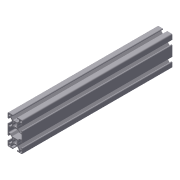
# Autodesk Inventor part: 30x60x2 in
Saved by Autodesk Inventor 2013 (Build 170138000, 138)
## iProperties
Created: 2011-07-21
Part Number: 30x60x2 in
Document SubType Name: Modeling
Designer: Dan Niemitalo
Density: 2.71 g/cm^3
Material: Aluminum-6061
Mass: 75.8168 g
Surface Area: 296.17 cm^2
Volume: 27.9767 cm^3
Author: Dan Niemitalo
Autodesk Inventor part; units mm, degrees
ref_plane "YZ Plane" through (0, 0, 0) normal (1, 0, 0) x (0, 1, 0)
ref_plane "XZ Plane" through (0, 0, 0) normal (0, 1, 0) x (-1, 0, 0)
ref_plane "XY Plane" through (0, 0, 0) normal (0, 0, 1) x (1, 0, 0)
sketch "3060" plane through (0, 0, 0) normal (0, 0, 1) x (1, 0, 0)
  line L0 (-0.1, 57.8) -> (3.3, 57.8)
  line L1 (-0.2, 59.8) -> (-0.2, 59.7)
  line L2 (-0.4, 59.5) -> (-0.5, 59.5)
  arc A0 (0, 60) -> (-0.2, 59.8) centre (0, 59.8) ccw
  arc A1 (-0.4, 59.5) -> (-0.2, 59.7) centre (-0.4, 59.7) ccw
  arc A2 (-0.5, 59.5) -> (-0.7, 59.3) centre (-0.5, 59.3) ccw
  line L3 (-0.7, 59.3) -> (-0.7, 58.4)
  arc A3 (-0.7, 58.4) -> (-0.1, 57.8) centre (-0.1, 58.4) ccw
  line L4 (-19.05, 49.05) -> (-18.15, 49.05)
  arc A4 (-19.25, 49.25) -> (-19.05, 49.05) centre (-19.05, 49.25) ccw
  line L5 (-19.25, 49.35) -> (-19.25, 49.25)
  arc A5 (-18.15, 49.05) -> (-17.55, 49.65) centre (-18.15, 49.65) ccw
  arc A6 (-19.25, 49.35) -> (-19.45, 49.55) centre (-19.45, 49.35) ccw
  line L6 (-19.55, 49.55) -> (-19.45, 49.55)
  arc A7 (-19.75, 49.75) -> (-19.55, 49.55) centre (-19.55, 49.75) ccw
  arc A8 (-17.35, 53.25) -> (-17.55, 53.05) centre (-17.35, 53.05) ccw
  line L7 (-17.35, 53.25) -> (-14.8828, 53.25)
  arc A9 (-18.45, 55.5) -> (-17.45, 54.5) centre (-17.45, 55.5) ccw
  line L8 (-19.75, 58) -> (-19.75, 49.75)
  line L9 (-17.55, 49.65) -> (-17.55, 53.05)
  arc A10 (-6.3501, 41.7194) -> (-3.1499, 41.7194) centre (-4.75, 45) ccw
  line L10 (0.5997, 38.4955) -> (-10.0997, 38.4955)
  arc A11 (-1.4694, 43.3999) -> (-1.4694, 46.6001) centre (-4.75, 45) ccw
  line L11 (-3.1499, 41.7194) -> (-1.5953, 40.4947)
  arc A12 (-1.5953, 40.4947) -> (-0.2316, 41.8641) centre (-4.75, 45) ccw
  line L12 (-0.2316, 41.8641) -> (-1.4694, 43.3999)
  line L13 (1.2545, 40.8784) -> (1.2545, 44.1)
  arc A13 (1.2545, 40.8784) -> (1.313, 40.737) centre (1.4545, 40.8784) ccw
  line L14 (-7.9047, 40.4947) -> (-6.3501, 41.7194)
  arc A14 (-9.2684, 41.8641) -> (-7.9047, 40.4947) centre (-4.75, 45) ccw
  line L15 (-8.0306, 43.3999) -> (-9.2684, 41.8641)
  arc A15 (-8.0306, 46.6001) -> (-8.0306, 43.3999) centre (-4.75, 45) ccw
  line L16 (-10.7545, 44.1) -> (-10.7545, 40.8784)
  arc A16 (-10.2926, 44.9) -> (-10.2926, 45.1) centre (-10.4658, 45) ccw
  line L17 (-10.2926, 44.9) -> (-10.7545, 44.1)
  arc A17 (-3.1499, 48.2806) -> (-6.3501, 48.2806) centre (-4.75, 45) ccw
  line L18 (-6.3501, 48.2806) -> (-7.9047, 49.5053)
  line L19 (-9.2684, 48.1359) -> (-8.0306, 46.6001)
  line L20 (-5.65, 51) -> (-8.8672, 51)
  arc A18 (-7.9047, 49.5053) -> (-9.2684, 48.1359) centre (-4.75, 45) ccw
  line L21 (-10.7545, 49.1216) -> (-10.7545, 45.9)
  arc A19 (-10.7545, 49.1216) -> (-10.813, 49.263) centre (-10.9545, 49.1216) ccw
  line L22 (-10.7545, 45.9) -> (-10.2926, 45.1)
  arc A20 (-0.2316, 48.1359) -> (-1.5953, 49.5053) centre (-4.75, 45) ccw
  line L23 (-1.4694, 46.6001) -> (-0.2316, 48.1359)
  arc A21 (-0.6328, 51) -> (-0.4914, 51.0586) centre (-0.6328, 51.2) ccw
  arc A22 (1.313, 49.263) -> (1.2545, 49.1216) centre (1.4545, 49.1216) ccw
  line L24 (1.313, 49.263) -> (5.2414, 53.1914)
  line L25 (3.4414, 54.9914) -> (-0.4914, 51.0586)
  arc A23 (-14.7414, 53.1914) -> (-14.8828, 53.25) centre (-14.8828, 53.05) ccw
  line L26 (-14.7414, 53.1914) -> (-10.813, 49.263)
  arc A24 (-13, 55.1328) -> (-12.9414, 54.9914) centre (-12.8, 55.1328) ccw
  arc A25 (-9.0086, 51.0586) -> (-8.8672, 51) centre (-8.8672, 51.2) ccw
  line L27 (-9.0086, 51.0586) -> (-12.9414, 54.9914)
  line L28 (-13, 55.1328) -> (-13, 57.6)
  arc A26 (-12.8, 57.8) -> (-13, 57.6) centre (-12.8, 57.6) ccw
  line L29 (-14.25, 55.5) -> (-14.25, 57.7)
  line L30 (-18.45, 57.7) -> (-18.45, 55.5)
  arc A27 (-17.45, 58.7) -> (-18.45, 57.7) centre (-17.45, 57.7) ccw
  arc A28 (-17.75, 60) -> (-19.75, 58) centre (-17.75, 58) ccw
  line L31 (-15.25, 58.7) -> (-17.45, 58.7)
  arc A29 (-14.25, 57.7) -> (-15.25, 58.7) centre (-15.25, 57.7) ccw
  line L32 (-12.8, 57.8) -> (-9.4, 57.8)
  arc A30 (-15.25, 54.5) -> (-14.25, 55.5) centre (-15.25, 55.5) ccw
  arc A31 (-9.4, 57.8) -> (-8.8, 58.4) centre (-9.4, 58.4) ccw
  line L33 (-9.5, 60) -> (-17.75, 60)
  line L34 (-9, 59.5) -> (-9.1, 59.5)
  line L35 (-8.8, 58.4) -> (-8.8, 59.3)
  arc A32 (-8.8, 59.3) -> (-9, 59.5) centre (-9, 59.3) ccw
  arc A33 (-9.3, 59.7) -> (-9.1, 59.5) centre (-9.1, 59.7) ccw
  line L36 (-9.3, 59.7) -> (-9.3, 59.8)
  arc A34 (-9.3, 59.8) -> (-9.5, 60) centre (-9.5, 59.8) ccw
  line L37 (-17.45, 54.5) -> (-15.25, 54.5)
  arc A35 (8.05, 53.05) -> (7.85, 53.25) centre (7.85, 53.05) ccw
  line L38 (8.05, 53.05) -> (8.05, 49.65)
  line L39 (10.25, 49.75) -> (10.25, 58)
  arc A36 (8.05, 49.65) -> (8.65, 49.05) centre (8.65, 49.65) ccw
  line L40 (8.65, 49.05) -> (9.55, 49.05)
  line L41 (9.75, 49.25) -> (9.75, 49.35)
  arc A37 (9.95, 49.55) -> (9.75, 49.35) centre (9.95, 49.35) ccw
  arc A38 (9.55, 49.05) -> (9.75, 49.25) centre (9.55, 49.25) ccw
  arc A39 (10.05, 49.55) -> (10.25, 49.75) centre (10.05, 49.75) ccw
  line L42 (9.95, 49.55) -> (10.05, 49.55)
  line L43 (5.75, 54.5) -> (7.95, 54.5)
  line L44 (7.95, 58.7) -> (5.75, 58.7)
  arc A40 (7.95, 54.5) -> (8.95, 55.5) centre (7.95, 55.5) ccw
  line L45 (8.95, 55.5) -> (8.95, 57.7)
  arc A41 (8.95, 57.7) -> (7.95, 58.7) centre (7.95, 57.7) ccw
  arc A42 (10.25, 58) -> (8.25, 60) centre (8.25, 58) ccw
  line L46 (8.25, 60) -> (0, 60)
  arc A43 (3.5, 57.6) -> (3.3, 57.8) centre (3.3, 57.6) ccw
  line L47 (3.5, 57.6) -> (3.5, 55.1328)
  arc A44 (3.4414, 54.9914) -> (3.5, 55.1328) centre (3.3, 55.1328) ccw
  arc A45 (5.75, 58.7) -> (4.75, 57.7) centre (5.75, 57.7) ccw
  line L48 (4.75, 57.7) -> (4.75, 55.5)
  arc A46 (4.75, 55.5) -> (5.75, 54.5) centre (5.75, 55.5) ccw
  arc A47 (5.3828, 53.25) -> (5.2414, 53.1914) centre (5.3828, 53.05) ccw
  line L49 (5.3828, 53.25) -> (7.85, 53.25)
  line L50 (1.2545, 44.1) -> (0.7926, 44.9)
  arc A48 (0.7926, 45.1) -> (0.7926, 44.9) centre (0.9658, 45) ccw
  line L51 (-4.8519, 50.5392) -> (-5.65, 51)
  arc A49 (-4.8519, 50.5392) -> (-4.6481, 50.5392) centre (-4.75, 50.7158) ccw
  line L52 (-3.85, 51) -> (-4.6481, 50.5392)
  line L53 (-1.5953, 49.5053) -> (-3.1499, 48.2806)
  line L54 (-0.6328, 51) -> (-3.85, 51)
  line L55 (1.2545, 45.9) -> (1.2545, 49.1216)
  line L56 (0.7926, 45.1) -> (1.2545, 45.9)
  arc A50 (-14.25, 4.5) -> (-15.25, 5.5) centre (-15.25, 4.5) ccw
  arc A51 (-14.8828, 6.75) -> (-14.7414, 6.8086) centre (-14.8828, 6.95) ccw
  line L57 (-15.25, 5.5) -> (-17.45, 5.5)
  line L58 (-14.8828, 6.75) -> (-17.35, 6.75)
  arc A52 (-19.75, 2) -> (-17.75, 0) centre (-17.75, 2) ccw
  arc A53 (-18.45, 2.3) -> (-17.45, 1.3) centre (-17.45, 2.3) ccw
  line L59 (-18.45, 4.5) -> (-18.45, 2.3)
  arc A54 (-17.45, 5.5) -> (-18.45, 4.5) centre (-17.45, 4.5) ccw
  arc A55 (-17.55, 6.95) -> (-17.35, 6.75) centre (-17.35, 6.95) ccw
  line L60 (-17.55, 6.95) -> (-17.55, 10.35)
  line L61 (-19.75, 10.25) -> (-19.75, 2)
  line L62 (0.7926, 15.1) -> (1.2545, 15.9)
  arc A56 (0.7926, 15.1) -> (0.7926, 14.9) centre (0.9658, 15) ccw
  line L63 (1.2545, 14.1) -> (0.7926, 14.9)
  line L64 (1.2545, 10.8784) -> (1.2545, 14.1)
  arc A57 (1.2545, 10.8784) -> (1.313, 10.737) centre (1.4545, 10.8784) ccw
  arc A58 (5.75, 5.5) -> (4.75, 4.5) centre (5.75, 4.5) ccw
  arc A59 (-0.4914, 8.9414) -> (-0.6328, 9) centre (-0.6328, 8.8) ccw
  line L65 (-0.4914, 8.9414) -> (3.4414, 5.0086)
  arc A60 (5.2414, 6.8086) -> (5.3828, 6.75) centre (5.3828, 6.95) ccw
  line L66 (7.95, 5.5) -> (5.75, 5.5)
  line L67 (7.85, 6.75) -> (5.3828, 6.75)
  line L68 (5.2414, 6.8086) -> (1.313, 10.737)
  arc A61 (3.5, 4.8672) -> (3.4414, 5.0086) centre (3.3, 4.8672) ccw
  line L69 (3.5, 4.8672) -> (3.5, 2.4)
  line L70 (0, 0) -> (8.25, 0)
  arc A62 (3.3, 2.2) -> (3.5, 2.4) centre (3.3, 2.4) ccw
  line L71 (3.3, 2.2) -> (-0.1, 2.2)
  arc A63 (-18.15, 19.05) -> (-17.55, 19.65) centre (-18.15, 19.65) ccw
  line L72 (-17.55, 19.65) -> (-17.55, 23.05)
  line L73 (-17.35, 23.25) -> (-14.8828, 23.25)
  arc A64 (-14.7414, 23.1914) -> (-14.8828, 23.25) centre (-14.8828, 23.05) ccw
  line L74 (-16.6, 24.9) -> (-14.7379, 24.9)
  line L75 (-14.7414, 23.1914) -> (-10.813, 19.263)
  arc A65 (-11.1604, 21.9438) -> (-10.0997, 21.5045) centre (-10.0997, 23.0045) ccw
  line L76 (-13.6772, 24.4607) -> (-11.1604, 21.9438)
  arc A66 (-13.6772, 24.4607) -> (-14.7379, 24.9) centre (-14.7379, 23.4) ccw
  arc A67 (-18.1, 26.4) -> (-16.6, 24.9) centre (-16.6, 26.4) ccw
  arc A68 (-17.35, 23.25) -> (-17.55, 23.05) centre (-17.35, 23.05) ccw
  arc A69 (-16.6, 35.1) -> (-18.1, 33.6) centre (-16.6, 33.6) ccw
  line L77 (-14.7379, 35.1) -> (-16.6, 35.1)
  arc A70 (-14.7379, 35.1) -> (-13.6772, 35.5393) centre (-14.7379, 36.6) ccw
  line L78 (-14.8828, 36.75) -> (-17.35, 36.75)
  arc A71 (-17.55, 36.95) -> (-17.35, 36.75) centre (-17.35, 36.95) ccw
  arc A72 (-14.8828, 36.75) -> (-14.7414, 36.8086) centre (-14.8828, 36.95) ccw
  line L79 (-11.1604, 38.0562) -> (-13.6772, 35.5393)
  arc A73 (-10.0997, 38.4955) -> (-11.1604, 38.0562) centre (-10.0997, 36.9955) ccw
  line L80 (-10.813, 40.737) -> (-14.7414, 36.8086)
  arc A74 (-10.813, 40.737) -> (-10.7545, 40.8784) centre (-10.9545, 40.8784) ccw
  arc A75 (-12.9414, 5.0086) -> (-13, 4.8672) centre (-12.8, 4.8672) ccw
  line L81 (-12.9414, 5.0086) -> (-9.0086, 8.9414)
  line L82 (-10.813, 10.737) -> (-14.7414, 6.8086)
  arc A76 (-10.813, 10.737) -> (-10.7545, 10.8784) centre (-10.9545, 10.8784) ccw
  line L83 (-14.25, 2.3) -> (-14.25, 4.5)
  line L84 (-13, 2.4) -> (-13, 4.8672)
  arc A77 (-13, 2.4) -> (-12.8, 2.2) centre (-12.8, 2.4) ccw
  line L85 (-19.45, 40.45) -> (-19.55, 40.45)
  arc A78 (-19.55, 40.45) -> (-19.75, 40.25) centre (-19.55, 40.25) ccw
  arc A79 (-17.55, 40.35) -> (-18.15, 40.95) centre (-18.15, 40.35) ccw
  arc A80 (-19.45, 40.45) -> (-19.25, 40.65) centre (-19.45, 40.65) ccw
  line L86 (-19.25, 40.75) -> (-19.25, 40.65)
  line L87 (-18.15, 40.95) -> (-19.05, 40.95)
  arc A81 (-19.05, 40.95) -> (-19.25, 40.75) centre (-19.05, 40.75) ccw
  line L88 (-17.55, 36.95) -> (-17.55, 40.35)
  arc A82 (10.25, 40.25) -> (10.05, 40.45) centre (10.05, 40.25) ccw
  line L89 (10.05, 40.45) -> (9.95, 40.45)
  line L90 (5.2414, 36.8086) -> (1.313, 40.737)
  line L91 (8.05, 40.35) -> (8.05, 36.95)
  arc A83 (8.65, 40.95) -> (8.05, 40.35) centre (8.65, 40.35) ccw
  line L92 (9.75, 40.65) -> (9.75, 40.75)
  line L93 (9.55, 40.95) -> (8.65, 40.95)
  arc A84 (9.75, 40.65) -> (9.95, 40.45) centre (9.95, 40.65) ccw
  arc A85 (9.75, 40.75) -> (9.55, 40.95) centre (9.55, 40.75) ccw
  arc A86 (7.1, 24.9) -> (8.6, 26.4) centre (7.1, 26.4) ccw
  line L94 (5.2379, 24.9) -> (7.1, 24.9)
  arc A87 (5.2379, 24.9) -> (4.1772, 24.4607) centre (5.2379, 23.4) ccw
  line L95 (5.3828, 23.25) -> (7.85, 23.25)
  arc A88 (5.3828, 23.25) -> (5.2414, 23.1914) centre (5.3828, 23.05) ccw
  arc A89 (8.05, 23.05) -> (7.85, 23.25) centre (7.85, 23.05) ccw
  line L96 (1.6604, 21.9438) -> (4.1772, 24.4607)
  arc A90 (0.5997, 21.5045) -> (1.6604, 21.9438) centre (0.5997, 23.0045) ccw
  line L97 (8.05, 23.05) -> (8.05, 19.65)
  line L98 (1.313, 19.263) -> (5.2414, 23.1914)
  arc A91 (1.313, 19.263) -> (1.2545, 19.1216) centre (1.4545, 19.1216) ccw
  arc A92 (8.05, 19.65) -> (8.65, 19.05) centre (8.65, 19.65) ccw
  line L99 (9.95, 19.55) -> (10.05, 19.55)
  arc A93 (10.05, 19.55) -> (10.25, 19.75) centre (10.05, 19.75) ccw
  arc A94 (9.95, 19.55) -> (9.75, 19.35) centre (9.95, 19.35) ccw
  line L100 (9.75, 19.25) -> (9.75, 19.35)
  arc A95 (9.55, 19.05) -> (9.75, 19.25) centre (9.55, 19.25) ccw
  line L101 (8.65, 19.05) -> (9.55, 19.05)
  line L102 (1.2545, 15.9) -> (1.2545, 19.1216)
  line L103 (-1.5953, 19.5053) -> (-3.1499, 18.2806)
  arc A96 (-0.2316, 18.1359) -> (-1.5953, 19.5053) centre (-4.75, 15) ccw
  arc A97 (-3.1499, 18.2806) -> (-6.3501, 18.2806) centre (-4.75, 15) ccw
  line L104 (-10.0997, 21.5045) -> (0.5997, 21.5045)
  line L105 (-1.4694, 16.6001) -> (-0.2316, 18.1359)
  line L106 (-19.75, 40.25) -> (-19.75, 19.75)
  line L107 (-18.1, 33.6) -> (-18.1, 26.4)
  arc A98 (-10.2926, 14.9) -> (-10.2926, 15.1) centre (-10.4658, 15) ccw
  line L108 (-19.05, 19.05) -> (-18.15, 19.05)
  line L109 (-19.25, 19.35) -> (-19.25, 19.25)
  arc A99 (-19.25, 19.35) -> (-19.45, 19.55) centre (-19.45, 19.35) ccw
  line L110 (-19.55, 19.55) -> (-19.45, 19.55)
  arc A100 (-19.75, 19.75) -> (-19.55, 19.55) centre (-19.55, 19.75) ccw
  arc A101 (-19.25, 19.25) -> (-19.05, 19.05) centre (-19.05, 19.25) ccw
  line L111 (-10.7545, 15.9) -> (-10.2926, 15.1)
  line L112 (-10.2926, 14.9) -> (-10.7545, 14.1)
  line L113 (-10.7545, 14.1) -> (-10.7545, 10.8784)
  line L114 (-7.9047, 10.4947) -> (-6.3501, 11.7194)
  arc A102 (-9.2684, 11.8641) -> (-7.9047, 10.4947) centre (-4.75, 15) ccw
  line L115 (-8.0306, 13.3999) -> (-9.2684, 11.8641)
  line L116 (-6.3501, 18.2806) -> (-7.9047, 19.5053)
  line L117 (-9.2684, 18.1359) -> (-8.0306, 16.6001)
  arc A103 (-7.9047, 19.5053) -> (-9.2684, 18.1359) centre (-4.75, 15) ccw
  line L118 (-10.7545, 19.1216) -> (-10.7545, 15.9)
  arc A104 (-10.7545, 19.1216) -> (-10.813, 19.263) centre (-10.9545, 19.1216) ccw
  arc A105 (-8.0306, 16.6001) -> (-8.0306, 13.3999) centre (-4.75, 15) ccw
  arc A106 (-1.5953, 10.4947) -> (-0.2316, 11.8641) centre (-4.75, 15) ccw
  line L119 (-3.1499, 11.7194) -> (-1.5953, 10.4947)
  line L120 (-3.85, 9) -> (-0.6328, 9)
  line L121 (-4.6481, 9.4608) -> (-3.85, 9)
  line L122 (-0.2316, 11.8641) -> (-1.4694, 13.3999)
  arc A107 (-1.4694, 13.3999) -> (-1.4694, 16.6001) centre (-4.75, 15) ccw
  arc A108 (-6.3501, 11.7194) -> (-3.1499, 11.7194) centre (-4.75, 15) ccw
  line L123 (-5.65, 9) -> (-4.8519, 9.4608)
  line L124 (-8.8672, 9) -> (-5.65, 9)
  arc A109 (-8.8672, 9) -> (-9.0086, 8.9414) centre (-8.8672, 8.8) ccw
  arc A110 (-4.6481, 9.4608) -> (-4.8519, 9.4608) centre (-4.75, 9.2842) ccw
  arc A111 (8.65, 10.95) -> (8.05, 10.35) centre (8.65, 10.35) ccw
  line L125 (9.55, 10.95) -> (8.65, 10.95)
  line L126 (10.05, 10.45) -> (9.95, 10.45)
  line L127 (9.75, 10.65) -> (9.75, 10.75)
  arc A112 (9.75, 10.65) -> (9.95, 10.45) centre (9.95, 10.65) ccw
  arc A113 (9.75, 10.75) -> (9.55, 10.95) centre (9.55, 10.75) ccw
  arc A114 (10.25, 10.25) -> (10.05, 10.45) centre (10.05, 10.25) ccw
  arc A115 (-17.55, 10.35) -> (-18.15, 10.95) centre (-18.15, 10.35) ccw
  line L128 (-18.15, 10.95) -> (-19.05, 10.95)
  line L129 (-19.25, 10.75) -> (-19.25, 10.65)
  arc A116 (-19.45, 10.45) -> (-19.25, 10.65) centre (-19.45, 10.65) ccw
  arc A117 (-19.05, 10.95) -> (-19.25, 10.75) centre (-19.05, 10.75) ccw
  arc A118 (-19.55, 10.45) -> (-19.75, 10.25) centre (-19.55, 10.25) ccw
  line L130 (-19.45, 10.45) -> (-19.55, 10.45)
  arc A119 (-8.8, 1.6) -> (-9.4, 2.2) centre (-9.4, 1.6) ccw
  line L131 (-9.4, 2.2) -> (-12.8, 2.2)
  line L132 (-17.45, 1.3) -> (-15.25, 1.3)
  arc A120 (-15.25, 1.3) -> (-14.25, 2.3) centre (-15.25, 2.3) ccw
  line L133 (-8.8, 0.7) -> (-8.8, 1.6)
  arc A121 (-9, 0.5) -> (-8.8, 0.7) centre (-9, 0.7) ccw
  line L134 (-9.1, 0.5) -> (-9, 0.5)
  arc A122 (-9.1, 0.5) -> (-9.3, 0.3) centre (-9.1, 0.3) ccw
  line L135 (-9.3, 0.2) -> (-9.3, 0.3)
  arc A123 (-9.5, 0) -> (-9.3, 0.2) centre (-9.5, 0.2) ccw
  line L136 (-17.75, 0) -> (-9.5, 0)
  arc A124 (-0.1, 2.2) -> (-0.7, 1.6) centre (-0.1, 1.6) ccw
  line L137 (-0.7, 1.6) -> (-0.7, 0.7)
  line L138 (-0.5, 0.5) -> (-0.4, 0.5)
  line L139 (-0.2, 0.3) -> (-0.2, 0.2)
  arc A125 (-0.7, 0.7) -> (-0.5, 0.5) centre (-0.5, 0.7) ccw
  arc A126 (-0.2, 0.2) -> (0, 0) centre (0, 0.2) ccw
  arc A127 (-0.2, 0.3) -> (-0.4, 0.5) centre (-0.4, 0.3) ccw
  line L140 (8.05, 10.35) -> (8.05, 6.95)
  arc A128 (7.85, 6.75) -> (8.05, 6.95) centre (7.85, 6.95) ccw
  line L141 (10.25, 2) -> (10.25, 10.25)
  arc A129 (8.95, 4.5) -> (7.95, 5.5) centre (7.95, 4.5) ccw
  line L142 (8.95, 2.3) -> (8.95, 4.5)
  arc A130 (7.95, 1.3) -> (8.95, 2.3) centre (7.95, 2.3) ccw
  arc A131 (8.25, 0) -> (10.25, 2) centre (8.25, 2) ccw
  line L143 (4.75, 4.5) -> (4.75, 2.3)
  line L144 (5.75, 1.3) -> (7.95, 1.3)
  arc A132 (4.75, 2.3) -> (5.75, 1.3) centre (5.75, 2.3) ccw
  line L145 (10.25, 19.75) -> (10.25, 40.25)
  line L146 (8.6, 26.4) -> (8.6, 33.6)
  arc A133 (8.6, 33.6) -> (7.1, 35.1) centre (7.1, 33.6) ccw
  line L147 (7.1, 35.1) -> (5.2379, 35.1)
  arc A134 (4.1772, 35.5393) -> (5.2379, 35.1) centre (5.2379, 36.6) ccw
  line L148 (7.85, 36.75) -> (5.3828, 36.75)
  arc A135 (7.85, 36.75) -> (8.05, 36.95) centre (7.85, 36.95) ccw
  line L149 (4.1772, 35.5393) -> (1.6604, 38.0562)
  arc A136 (1.6604, 38.0562) -> (0.5997, 38.4955) centre (0.5997, 36.9955) ccw
  arc A137 (5.2414, 36.8086) -> (5.3828, 36.75) centre (5.3828, 36.95) ccw
  point P0 (-4.75, 30)
  point P1 (-4.75, 30)
sketch "Sketch1" plane through (0, 0, 0) normal (0, 0, 1) x (1, 0, 0)
  line L0 (4.65, 27.8) -> (8.05, 27.8)
  line L1 (4.55, 29.8) -> (4.55, 29.7)
  line L2 (4.35, 29.5) -> (4.25, 29.5)
  arc A0 (4.75, 30) -> (4.55, 29.8) centre (4.75, 29.8) ccw
  arc A1 (4.35, 29.5) -> (4.55, 29.7) centre (4.35, 29.7) ccw
  arc A2 (4.25, 29.5) -> (4.05, 29.3) centre (4.25, 29.3) ccw
  line L3 (4.05, 29.3) -> (4.05, 28.4)
  arc A3 (4.05, 28.4) -> (4.65, 27.8) centre (4.65, 28.4) ccw
  line L4 (-14.3, 19.05) -> (-13.4, 19.05)
  arc A4 (-14.5, 19.25) -> (-14.3, 19.05) centre (-14.3, 19.25) ccw
  line L5 (-14.5, 19.35) -> (-14.5, 19.25)
  arc A5 (-13.4, 19.05) -> (-12.8, 19.65) centre (-13.4, 19.65) ccw
  arc A6 (-14.5, 19.35) -> (-14.7, 19.55) centre (-14.7, 19.35) ccw
  line L6 (-14.8, 19.55) -> (-14.7, 19.55)
  arc A7 (-15, 19.75) -> (-14.8, 19.55) centre (-14.8, 19.75) ccw
  arc A8 (-12.6, 23.25) -> (-12.8, 23.05) centre (-12.6, 23.05) ccw
  line L7 (-12.6, 23.25) -> (-10.1328, 23.25)
  arc A9 (-13.7, 25.5) -> (-12.7, 24.5) centre (-12.7, 25.5) ccw
  line L8 (-15, 28) -> (-15, 19.75)
  line L9 (-12.8, 19.65) -> (-12.8, 23.05)
  arc A10 (-1.6001, 11.7194) -> (1.6001, 11.7194) centre (0, 15) ccw
  line L10 (5.3497, 8.4955) -> (-5.3497, 8.4955)
  arc A11 (3.2806, 13.3999) -> (3.2806, 16.6001) centre (0, 15) ccw
  line L11 (1.6001, 11.7194) -> (3.1547, 10.4947)
  arc A12 (3.1547, 10.4947) -> (4.5184, 11.8641) centre (0, 15) ccw
  line L12 (4.5184, 11.8641) -> (3.2806, 13.3999)
  line L13 (6.0045, 10.8784) -> (6.0045, 14.1)
  arc A13 (6.0045, 10.8784) -> (6.063, 10.737) centre (6.2045, 10.8784) ccw
  line L14 (-3.1547, 10.4947) -> (-1.6001, 11.7194)
  arc A14 (-4.5184, 11.8641) -> (-3.1547, 10.4947) centre (0, 15) ccw
  line L15 (-3.2806, 13.3999) -> (-4.5184, 11.8641)
  arc A15 (-3.2806, 16.6001) -> (-3.2806, 13.3999) centre (0, 15) ccw
  line L16 (-6.0045, 14.1) -> (-6.0045, 10.8784)
  arc A16 (-5.5426, 14.9) -> (-5.5426, 15.1) centre (-5.7158, 15) ccw
  line L17 (-5.5426, 14.9) -> (-6.0045, 14.1)
  arc A17 (1.6001, 18.2806) -> (-1.6001, 18.2806) centre (0, 15) ccw
  line L18 (-1.6001, 18.2806) -> (-3.1547, 19.5053)
  line L19 (-4.5184, 18.1359) -> (-3.2806, 16.6001)
  line L20 (-0.9, 21) -> (-4.1172, 21)
  arc A18 (-3.1547, 19.5053) -> (-4.5184, 18.1359) centre (0, 15) ccw
  line L21 (-6.0045, 19.1216) -> (-6.0045, 15.9)
  arc A19 (-6.0045, 19.1216) -> (-6.063, 19.263) centre (-6.2045, 19.1216) ccw
  line L22 (-6.0045, 15.9) -> (-5.5426, 15.1)
  arc A20 (4.5184, 18.1359) -> (3.1547, 19.5053) centre (0, 15) ccw
  line L23 (3.2806, 16.6001) -> (4.5184, 18.1359)
  arc A21 (4.1172, 21) -> (4.2586, 21.0586) centre (4.1172, 21.2) ccw
  arc A22 (6.063, 19.263) -> (6.0045, 19.1216) centre (6.2045, 19.1216) ccw
  line L24 (6.063, 19.263) -> (9.9914, 23.1914)
  line L25 (8.1914, 24.9914) -> (4.2586, 21.0586)
  arc A23 (-9.9914, 23.1914) -> (-10.1328, 23.25) centre (-10.1328, 23.05) ccw
  line L26 (-9.9914, 23.1914) -> (-6.063, 19.263)
  arc A24 (-8.25, 25.1328) -> (-8.1914, 24.9914) centre (-8.05, 25.1328) ccw
  arc A25 (-4.2586, 21.0586) -> (-4.1172, 21) centre (-4.1172, 21.2) ccw
  line L27 (-4.2586, 21.0586) -> (-8.1914, 24.9914)
  line L28 (-8.25, 25.1328) -> (-8.25, 27.6)
  arc A26 (-8.05, 27.8) -> (-8.25, 27.6) centre (-8.05, 27.6) ccw
  line L29 (-9.5, 25.5) -> (-9.5, 27.7)
  line L30 (-13.7, 27.7) -> (-13.7, 25.5)
  arc A27 (-12.7, 28.7) -> (-13.7, 27.7) centre (-12.7, 27.7) ccw
  arc A28 (-13, 30) -> (-15, 28) centre (-13, 28) ccw
  line L31 (-10.5, 28.7) -> (-12.7, 28.7)
  arc A29 (-9.5, 27.7) -> (-10.5, 28.7) centre (-10.5, 27.7) ccw
  line L32 (-8.05, 27.8) -> (-4.65, 27.8)
  arc A30 (-10.5, 24.5) -> (-9.5, 25.5) centre (-10.5, 25.5) ccw
  arc A31 (-4.65, 27.8) -> (-4.05, 28.4) centre (-4.65, 28.4) ccw
  line L33 (-4.75, 30) -> (-13, 30)
  line L34 (-4.25, 29.5) -> (-4.35, 29.5)
  line L35 (-4.05, 28.4) -> (-4.05, 29.3)
  arc A32 (-4.05, 29.3) -> (-4.25, 29.5) centre (-4.25, 29.3) ccw
  arc A33 (-4.55, 29.7) -> (-4.35, 29.5) centre (-4.35, 29.7) ccw
  line L36 (-4.55, 29.7) -> (-4.55, 29.8)
  arc A34 (-4.55, 29.8) -> (-4.75, 30) centre (-4.75, 29.8) ccw
  line L37 (-12.7, 24.5) -> (-10.5, 24.5)
  arc A35 (12.8, 23.05) -> (12.6, 23.25) centre (12.6, 23.05) ccw
  line L38 (12.8, 23.05) -> (12.8, 19.65)
  line L39 (15, 19.75) -> (15, 28)
  arc A36 (12.8, 19.65) -> (13.4, 19.05) centre (13.4, 19.65) ccw
  line L40 (13.4, 19.05) -> (14.3, 19.05)
  line L41 (14.5, 19.25) -> (14.5, 19.35)
  arc A37 (14.7, 19.55) -> (14.5, 19.35) centre (14.7, 19.35) ccw
  arc A38 (14.3, 19.05) -> (14.5, 19.25) centre (14.3, 19.25) ccw
  arc A39 (14.8, 19.55) -> (15, 19.75) centre (14.8, 19.75) ccw
  line L42 (14.7, 19.55) -> (14.8, 19.55)
  line L43 (10.5, 24.5) -> (12.7, 24.5)
  line L44 (12.7, 28.7) -> (10.5, 28.7)
  arc A40 (12.7, 24.5) -> (13.7, 25.5) centre (12.7, 25.5) ccw
  line L45 (13.7, 25.5) -> (13.7, 27.7)
  arc A41 (13.7, 27.7) -> (12.7, 28.7) centre (12.7, 27.7) ccw
  arc A42 (15, 28) -> (13, 30) centre (13, 28) ccw
  line L46 (13, 30) -> (4.75, 30)
  arc A43 (8.25, 27.6) -> (8.05, 27.8) centre (8.05, 27.6) ccw
  line L47 (8.25, 27.6) -> (8.25, 25.1328)
  arc A44 (8.1914, 24.9914) -> (8.25, 25.1328) centre (8.05, 25.1328) ccw
  arc A45 (10.5, 28.7) -> (9.5, 27.7) centre (10.5, 27.7) ccw
  line L48 (9.5, 27.7) -> (9.5, 25.5)
  arc A46 (9.5, 25.5) -> (10.5, 24.5) centre (10.5, 25.5) ccw
  arc A47 (10.1328, 23.25) -> (9.9914, 23.1914) centre (10.1328, 23.05) ccw
  line L49 (10.1328, 23.25) -> (12.6, 23.25)
  line L50 (6.0045, 14.1) -> (5.5426, 14.9)
  arc A48 (5.5426, 15.1) -> (5.5426, 14.9) centre (5.7158, 15) ccw
  line L51 (-0.1019, 20.5392) -> (-0.9, 21)
  arc A49 (-0.1019, 20.5392) -> (0.1019, 20.5392) centre (0, 20.7158) ccw
  line L52 (0.9, 21) -> (0.1019, 20.5392)
  line L53 (3.1547, 19.5053) -> (1.6001, 18.2806)
  line L54 (4.1172, 21) -> (0.9, 21)
  line L55 (6.0045, 15.9) -> (6.0045, 19.1216)
  line L56 (5.5426, 15.1) -> (6.0045, 15.9)
  arc A50 (-9.5, -25.5) -> (-10.5, -24.5) centre (-10.5, -25.5) ccw
  arc A51 (-10.1328, -23.25) -> (-9.9914, -23.1914) centre (-10.1328, -23.05) ccw
  line L57 (-10.5, -24.5) -> (-12.7, -24.5)
  line L58 (-10.1328, -23.25) -> (-12.6, -23.25)
  arc A52 (-15, -28) -> (-13, -30) centre (-13, -28) ccw
  arc A53 (-13.7, -27.7) -> (-12.7, -28.7) centre (-12.7, -27.7) ccw
  line L59 (-13.7, -25.5) -> (-13.7, -27.7)
  arc A54 (-12.7, -24.5) -> (-13.7, -25.5) centre (-12.7, -25.5) ccw
  arc A55 (-12.8, -23.05) -> (-12.6, -23.25) centre (-12.6, -23.05) ccw
  line L60 (-12.8, -23.05) -> (-12.8, -19.65)
  line L61 (-15, -19.75) -> (-15, -28)
  line L62 (5.5426, -14.9) -> (6.0045, -14.1)
  arc A56 (5.5426, -14.9) -> (5.5426, -15.1) centre (5.7158, -15) ccw
  line L63 (6.0045, -15.9) -> (5.5426, -15.1)
  line L64 (6.0045, -19.1216) -> (6.0045, -15.9)
  arc A57 (6.0045, -19.1216) -> (6.063, -19.263) centre (6.2045, -19.1216) ccw
  arc A58 (10.5, -24.5) -> (9.5, -25.5) centre (10.5, -25.5) ccw
  arc A59 (4.2586, -21.0586) -> (4.1172, -21) centre (4.1172, -21.2) ccw
  line L65 (4.2586, -21.0586) -> (8.1914, -24.9914)
  arc A60 (9.9914, -23.1914) -> (10.1328, -23.25) centre (10.1328, -23.05) ccw
  line L66 (12.7, -24.5) -> (10.5, -24.5)
  line L67 (12.6, -23.25) -> (10.1328, -23.25)
  line L68 (9.9914, -23.1914) -> (6.063, -19.263)
  arc A61 (8.25, -25.1328) -> (8.1914, -24.9914) centre (8.05, -25.1328) ccw
  line L69 (8.25, -25.1328) -> (8.25, -27.6)
  line L70 (4.75, -30) -> (13, -30)
  arc A62 (8.05, -27.8) -> (8.25, -27.6) centre (8.05, -27.6) ccw
  line L71 (8.05, -27.8) -> (4.65, -27.8)
  arc A63 (-13.4, -10.95) -> (-12.8, -10.35) centre (-13.4, -10.35) ccw
  line L72 (-12.8, -10.35) -> (-12.8, -6.95)
  line L73 (-12.6, -6.75) -> (-10.1328, -6.75)
  arc A64 (-9.9914, -6.8086) -> (-10.1328, -6.75) centre (-10.1328, -6.95) ccw
  line L74 (-11.85, -5.1) -> (-9.9879, -5.1)
  line L75 (-9.9914, -6.8086) -> (-6.063, -10.737)
  arc A65 (-6.4104, -8.0562) -> (-5.3497, -8.4955) centre (-5.3497, -6.9955) ccw
  line L76 (-8.9272, -5.5393) -> (-6.4104, -8.0562)
  arc A66 (-8.9272, -5.5393) -> (-9.9879, -5.1) centre (-9.9879, -6.6) ccw
  arc A67 (-13.35, -3.6) -> (-11.85, -5.1) centre (-11.85, -3.6) ccw
  arc A68 (-12.6, -6.75) -> (-12.8, -6.95) centre (-12.6, -6.95) ccw
  arc A69 (-11.85, 5.1) -> (-13.35, 3.6) centre (-11.85, 3.6) ccw
  line L77 (-9.9879, 5.1) -> (-11.85, 5.1)
  arc A70 (-9.9879, 5.1) -> (-8.9272, 5.5393) centre (-9.9879, 6.6) ccw
  line L78 (-10.1328, 6.75) -> (-12.6, 6.75)
  arc A71 (-12.8, 6.95) -> (-12.6, 6.75) centre (-12.6, 6.95) ccw
  arc A72 (-10.1328, 6.75) -> (-9.9914, 6.8086) centre (-10.1328, 6.95) ccw
  line L79 (-6.4104, 8.0562) -> (-8.9272, 5.5393)
  arc A73 (-5.3497, 8.4955) -> (-6.4104, 8.0562) centre (-5.3497, 6.9955) ccw
  line L80 (-6.063, 10.737) -> (-9.9914, 6.8086)
  arc A74 (-6.063, 10.737) -> (-6.0045, 10.8784) centre (-6.2045, 10.8784) ccw
  arc A75 (-8.1914, -24.9914) -> (-8.25, -25.1328) centre (-8.05, -25.1328) ccw
  line L81 (-8.1914, -24.9914) -> (-4.2586, -21.0586)
  line L82 (-6.063, -19.263) -> (-9.9914, -23.1914)
  arc A76 (-6.063, -19.263) -> (-6.0045, -19.1216) centre (-6.2045, -19.1216) ccw
  line L83 (-9.5, -27.7) -> (-9.5, -25.5)
  line L84 (-8.25, -27.6) -> (-8.25, -25.1328)
  arc A77 (-8.25, -27.6) -> (-8.05, -27.8) centre (-8.05, -27.6) ccw
  line L85 (-14.7, 10.45) -> (-14.8, 10.45)
  arc A78 (-14.8, 10.45) -> (-15, 10.25) centre (-14.8, 10.25) ccw
  arc A79 (-12.8, 10.35) -> (-13.4, 10.95) centre (-13.4, 10.35) ccw
  arc A80 (-14.7, 10.45) -> (-14.5, 10.65) centre (-14.7, 10.65) ccw
  line L86 (-14.5, 10.75) -> (-14.5, 10.65)
  line L87 (-13.4, 10.95) -> (-14.3, 10.95)
  arc A81 (-14.3, 10.95) -> (-14.5, 10.75) centre (-14.3, 10.75) ccw
  line L88 (-12.8, 6.95) -> (-12.8, 10.35)
  arc A82 (15, 10.25) -> (14.8, 10.45) centre (14.8, 10.25) ccw
  line L89 (14.8, 10.45) -> (14.7, 10.45)
  line L90 (9.9914, 6.8086) -> (6.063, 10.737)
  line L91 (12.8, 10.35) -> (12.8, 6.95)
  arc A83 (13.4, 10.95) -> (12.8, 10.35) centre (13.4, 10.35) ccw
  line L92 (14.5, 10.65) -> (14.5, 10.75)
  line L93 (14.3, 10.95) -> (13.4, 10.95)
  arc A84 (14.5, 10.65) -> (14.7, 10.45) centre (14.7, 10.65) ccw
  arc A85 (14.5, 10.75) -> (14.3, 10.95) centre (14.3, 10.75) ccw
  arc A86 (11.85, -5.1) -> (13.35, -3.6) centre (11.85, -3.6) ccw
  line L94 (9.9879, -5.1) -> (11.85, -5.1)
  arc A87 (9.9879, -5.1) -> (8.9272, -5.5393) centre (9.9879, -6.6) ccw
  line L95 (10.1328, -6.75) -> (12.6, -6.75)
  arc A88 (10.1328, -6.75) -> (9.9914, -6.8086) centre (10.1328, -6.95) ccw
  arc A89 (12.8, -6.95) -> (12.6, -6.75) centre (12.6, -6.95) ccw
  line L96 (6.4104, -8.0562) -> (8.9272, -5.5393)
  arc A90 (5.3497, -8.4955) -> (6.4104, -8.0562) centre (5.3497, -6.9955) ccw
  line L97 (12.8, -6.95) -> (12.8, -10.35)
  line L98 (6.063, -10.737) -> (9.9914, -6.8086)
  arc A91 (6.063, -10.737) -> (6.0045, -10.8784) centre (6.2045, -10.8784) ccw
  arc A92 (12.8, -10.35) -> (13.4, -10.95) centre (13.4, -10.35) ccw
  line L99 (14.7, -10.45) -> (14.8, -10.45)
  arc A93 (14.8, -10.45) -> (15, -10.25) centre (14.8, -10.25) ccw
  arc A94 (14.7, -10.45) -> (14.5, -10.65) centre (14.7, -10.65) ccw
  line L100 (14.5, -10.75) -> (14.5, -10.65)
  arc A95 (14.3, -10.95) -> (14.5, -10.75) centre (14.3, -10.75) ccw
  line L101 (13.4, -10.95) -> (14.3, -10.95)
  line L102 (6.0045, -14.1) -> (6.0045, -10.8784)
  line L103 (3.1547, -10.4947) -> (1.6001, -11.7194)
  arc A96 (4.5184, -11.8641) -> (3.1547, -10.4947) centre (0, -15) ccw
  arc A97 (1.6001, -11.7194) -> (-1.6001, -11.7194) centre (0, -15) ccw
  line L104 (-5.3497, -8.4955) -> (5.3497, -8.4955)
  line L105 (3.2806, -13.3999) -> (4.5184, -11.8641)
  line L106 (-15, 10.25) -> (-15, -10.25)
  line L107 (-13.35, 3.6) -> (-13.35, -3.6)
  arc A98 (-5.5426, -15.1) -> (-5.5426, -14.9) centre (-5.7158, -15) ccw
  line L108 (-14.3, -10.95) -> (-13.4, -10.95)
  line L109 (-14.5, -10.65) -> (-14.5, -10.75)
  arc A99 (-14.5, -10.65) -> (-14.7, -10.45) centre (-14.7, -10.65) ccw
  line L110 (-14.8, -10.45) -> (-14.7, -10.45)
  arc A100 (-15, -10.25) -> (-14.8, -10.45) centre (-14.8, -10.25) ccw
  arc A101 (-14.5, -10.75) -> (-14.3, -10.95) centre (-14.3, -10.75) ccw
  line L111 (-6.0045, -14.1) -> (-5.5426, -14.9)
  line L112 (-5.5426, -15.1) -> (-6.0045, -15.9)
  line L113 (-6.0045, -15.9) -> (-6.0045, -19.1216)
  line L114 (-3.1547, -19.5053) -> (-1.6001, -18.2806)
  arc A102 (-4.5184, -18.1359) -> (-3.1547, -19.5053) centre (0, -15) ccw
  line L115 (-3.2806, -16.6001) -> (-4.5184, -18.1359)
  line L116 (-1.6001, -11.7194) -> (-3.1547, -10.4947)
  line L117 (-4.5184, -11.8641) -> (-3.2806, -13.3999)
  arc A103 (-3.1547, -10.4947) -> (-4.5184, -11.8641) centre (0, -15) ccw
  line L118 (-6.0045, -10.8784) -> (-6.0045, -14.1)
  arc A104 (-6.0045, -10.8784) -> (-6.063, -10.737) centre (-6.2045, -10.8784) ccw
  arc A105 (-3.2806, -13.3999) -> (-3.2806, -16.6001) centre (0, -15) ccw
  arc A106 (3.1547, -19.5053) -> (4.5184, -18.1359) centre (0, -15) ccw
  line L119 (1.6001, -18.2806) -> (3.1547, -19.5053)
  line L120 (0.9, -21) -> (4.1172, -21)
  line L121 (0.1019, -20.5392) -> (0.9, -21)
  line L122 (4.5184, -18.1359) -> (3.2806, -16.6001)
  arc A107 (3.2806, -16.6001) -> (3.2806, -13.3999) centre (0, -15) ccw
  arc A108 (-1.6001, -18.2806) -> (1.6001, -18.2806) centre (0, -15) ccw
  line L123 (-0.9, -21) -> (-0.1019, -20.5392)
  line L124 (-4.1172, -21) -> (-0.9, -21)
  arc A109 (-4.1172, -21) -> (-4.2586, -21.0586) centre (-4.1172, -21.2) ccw
  arc A110 (0.1019, -20.5392) -> (-0.1019, -20.5392) centre (0, -20.7158) ccw
  arc A111 (13.4, -19.05) -> (12.8, -19.65) centre (13.4, -19.65) ccw
  line L125 (14.3, -19.05) -> (13.4, -19.05)
  line L126 (14.8, -19.55) -> (14.7, -19.55)
  line L127 (14.5, -19.35) -> (14.5, -19.25)
  arc A112 (14.5, -19.35) -> (14.7, -19.55) centre (14.7, -19.35) ccw
  arc A113 (14.5, -19.25) -> (14.3, -19.05) centre (14.3, -19.25) ccw
  arc A114 (15, -19.75) -> (14.8, -19.55) centre (14.8, -19.75) ccw
  arc A115 (-12.8, -19.65) -> (-13.4, -19.05) centre (-13.4, -19.65) ccw
  line L128 (-13.4, -19.05) -> (-14.3, -19.05)
  line L129 (-14.5, -19.25) -> (-14.5, -19.35)
  arc A116 (-14.7, -19.55) -> (-14.5, -19.35) centre (-14.7, -19.35) ccw
  arc A117 (-14.3, -19.05) -> (-14.5, -19.25) centre (-14.3, -19.25) ccw
  arc A118 (-14.8, -19.55) -> (-15, -19.75) centre (-14.8, -19.75) ccw
  line L130 (-14.7, -19.55) -> (-14.8, -19.55)
  arc A119 (-4.05, -28.4) -> (-4.65, -27.8) centre (-4.65, -28.4) ccw
  line L131 (-4.65, -27.8) -> (-8.05, -27.8)
  line L132 (-12.7, -28.7) -> (-10.5, -28.7)
  arc A120 (-10.5, -28.7) -> (-9.5, -27.7) centre (-10.5, -27.7) ccw
  line L133 (-4.05, -29.3) -> (-4.05, -28.4)
  arc A121 (-4.25, -29.5) -> (-4.05, -29.3) centre (-4.25, -29.3) ccw
  line L134 (-4.35, -29.5) -> (-4.25, -29.5)
  arc A122 (-4.35, -29.5) -> (-4.55, -29.7) centre (-4.35, -29.7) ccw
  line L135 (-4.55, -29.8) -> (-4.55, -29.7)
  arc A123 (-4.75, -30) -> (-4.55, -29.8) centre (-4.75, -29.8) ccw
  line L136 (-13, -30) -> (-4.75, -30)
  arc A124 (4.65, -27.8) -> (4.05, -28.4) centre (4.65, -28.4) ccw
  line L137 (4.05, -28.4) -> (4.05, -29.3)
  line L138 (4.25, -29.5) -> (4.35, -29.5)
  line L139 (4.55, -29.7) -> (4.55, -29.8)
  arc A125 (4.05, -29.3) -> (4.25, -29.5) centre (4.25, -29.3) ccw
  arc A126 (4.55, -29.8) -> (4.75, -30) centre (4.75, -29.8) ccw
  arc A127 (4.55, -29.7) -> (4.35, -29.5) centre (4.35, -29.7) ccw
  line L140 (12.8, -19.65) -> (12.8, -23.05)
  arc A128 (12.6, -23.25) -> (12.8, -23.05) centre (12.6, -23.05) ccw
  line L141 (15, -28) -> (15, -19.75)
  arc A129 (13.7, -25.5) -> (12.7, -24.5) centre (12.7, -25.5) ccw
  line L142 (13.7, -27.7) -> (13.7, -25.5)
  arc A130 (12.7, -28.7) -> (13.7, -27.7) centre (12.7, -27.7) ccw
  arc A131 (13, -30) -> (15, -28) centre (13, -28) ccw
  line L143 (9.5, -25.5) -> (9.5, -27.7)
  line L144 (10.5, -28.7) -> (12.7, -28.7)
  arc A132 (9.5, -27.7) -> (10.5, -28.7) centre (10.5, -27.7) ccw
  line L145 (15, -10.25) -> (15, 10.25)
  line L146 (13.35, -3.6) -> (13.35, 3.6)
  arc A133 (13.35, 3.6) -> (11.85, 5.1) centre (11.85, 3.6) ccw
  line L147 (11.85, 5.1) -> (9.9879, 5.1)
  arc A134 (8.9272, 5.5393) -> (9.9879, 5.1) centre (9.9879, 6.6) ccw
  line L148 (12.6, 6.75) -> (10.1328, 6.75)
  arc A135 (12.6, 6.75) -> (12.8, 6.95) centre (12.6, 6.95) ccw
  line L149 (8.9272, 5.5393) -> (6.4104, 8.0562)
  arc A136 (6.4104, 8.0562) -> (5.3497, 8.4955) centre (5.3497, 6.9955) ccw
  arc A137 (9.9914, 6.8086) -> (10.1328, 6.75) centre (10.1328, 6.95) ccw
  point P0 (0, 0)
  point P1 (-13.35, 0)
  point P2 (0, 8.4955)
  constraints: 1 horizontal alignment, 1 vertical alignment, 2 other
extrude "Extrusion1" add sketch "Sketch1" along normal mid plane 304.8
body "Solid1"
